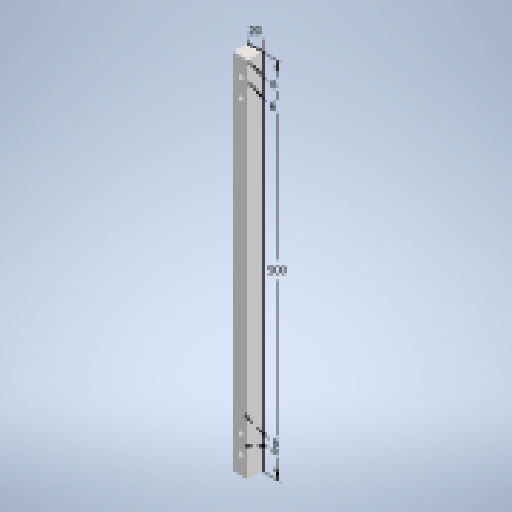
# Autodesk Inventor part: DOF11
Saved by Autodesk Inventor 2024 (Build 280153000, 153)
## iProperties
Created: 2024-10-17
Part Number: DOF11
Material: 一般
Document SubType Name: Modeling
Designer: jerry
Density: 1 g/cm^3
Appearance: 預設
Author: jerry
Autodesk Inventor part; units mm, degrees
ref_plane "YZ Plane" through (0, 0, 0) normal (1, 0, 0) x (0, 1, 0)
ref_plane "XZ Plane" through (0, 0, 0) normal (0, 1, 0) x (-1, 0, 0)
ref_plane "XY Plane" through (0, 0, 0) normal (0, 0, 1) x (1, 0, 0)
sketch "草圖1" plane through (0, 0, 0) normal (0, 0, 1) x (1, 0, 0)
  line L0 (-10, -250) -> (10, -250)
  line L1 (10, -250) -> (10, 250)
  line L2 (10, 250) -> (-10, 250)
  line L3 (-10, 250) -> (-10, -250)
  line L4 (-10, -250) -> (10, 250) construction
  line L5 (10, -250) -> (-10, 250) construction
  circle A0 centre (0, 225) radius 3
  circle A1 centre (0, 200) radius 3
  circle A2 centre (0, -200) radius 3
  circle A3 centre (0, -225) radius 3
  circle A4 centre (0, -175) radius 3
  circle A5 centre (0, 175) radius 3
  point P0 (0, 0)
  dimension "d0" = 20
  dimension "d1" = 500
  dimension "d6" = 6
  dimension "d7" = 6
  dimension "d10" = 6
  dimension "d11" = 6
  dimension "d15" = 6
  dimension "d17" = 6
  constraints: 12 end point, 6 centre point, 2 midpoint, 2 parallel, 1 horizontal, 1 perpendicular
  measures "d0" distance of L2.end L1.end
  measures "d1" distance of L1.end L0.end
  measures "d6" diameter of A0
  measures "d7" diameter of A1
  measures "d10" diameter of A2
  measures "d11" diameter of A3
  measures "d15" diameter of A4
  measures "d17" diameter of A5
extrude "擠出1" add sketch "草圖1" along normal blind 20 contours L3 L2 L1 L0 | A0 | A1 | A2 | A3 | A4 | A5
extrude "擠出2" cut sketch "草圖1" along normal blind 20 contours A0 | A1 | A2 | A3 | A4 | A5
